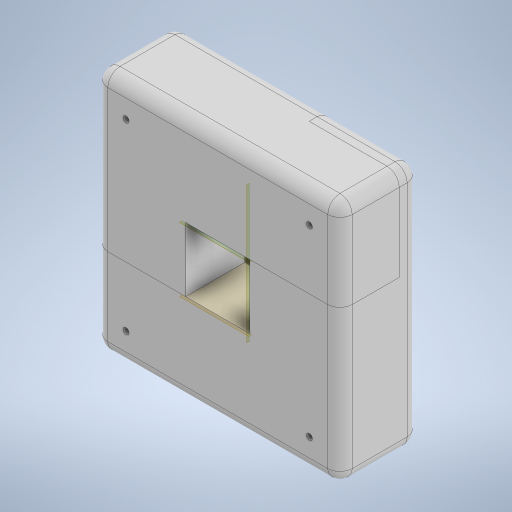
# Autodesk Inventor part: BGO-holder-C-conector
Saved by Autodesk Inventor 2023 (Build 270158000, 158)
## iProperties
Created: 2023-12-01
Part Number: BGO-holder-C-conector
Material: Generic
Document SubType Name: Modeling
Designer: AxLab
Density: 1 g/cm^3
Appearance: Default
Author: AxLab
Autodesk Inventor part; units mm, degrees
ref_plane "YZ Plane" through (0, 0, 0) normal (1, 0, 0) x (0, 1, 0)
ref_plane "XZ Plane" through (0, 0, 0) normal (0, 1, 0) x (-1, 0, 0)
ref_plane "XY Plane" through (0, 0, 0) normal (0, 0, 1) x (1, 0, 0)
sketch "Sketch1" plane through (0, 0, 0) normal (0, 0, 1) x (1, 0, 0)
  line L0 (-20, -20) -> (20, -20)
  line L1 (20, -20) -> (20, 20)
  line L2 (20, 20) -> (-20, 20)
  line L3 (-20, 20) -> (-20, -20)
  line L4 (-20, -20) -> (20, 20) construction
  line L5 (20, -20) -> (-20, 20) construction
  point P0 (0, 0)
  dimension "d0" = 40
  dimension "d1" = 40
  constraints: 12 end point, 2 midpoint, 2 parallel, 1 horizontal, 1 perpendicular
  measures "d0" distance of L2.end L1.end
  measures "d1" distance of L1.end L0.end
extrude "Extrusion1" add sketch "Sketch1" along normal blind 13
sketch "Sketch2" plane through (0, 0, 13) normal (0, 0, 1) x (1, 0, 0)
  line L0 (5.25, -5.25) -> (-5.25, -5.25)
  line L1 (-5.25, -5.25) -> (-5.25, 5.25)
  line L2 (-5.25, 5.25) -> (5.25, 5.25)
  line L3 (5.25, 5.25) -> (5.25, -5.25)
  line L4 (5.25, -5.25) -> (-5.25, 5.25) construction
  line L5 (-5.25, -5.25) -> (5.25, 5.25) construction
  point P0 (0, 0)
  dimension "d4" = 10.5
  dimension "d5" = 10.5
  constraints: 12 end point, 2 midpoint, 2 parallel, 1 horizontal, 1 perpendicular
  measures "d4" distance of L1.end L2.end
  measures "d5" distance of L0.end L1.end
extrude "Extrusion2" cut sketch "Sketch2" against normal blind 9.7
sketch "Sketch3" plane through (0, 0, 13) normal (0, 0, 1) x (1, 0, 0)
  line L0 (-20, 20) -> (-20, -20) projected
  line L1 (-20, 20) -> (-15, 20)
  line L2 (-15, 20) -> (-15, 15)
  line L3 (-15, 15) -> (-20, 15)
  line L4 (-20, 15) -> (-20, 20)
  circle A0 centre (-15, 15) radius 0.5
  point P0 (0, 0)
  dimension "d8" = 5
  dimension "d9" = 5
  dimension "d10" = 1
  constraints: 8 end point, 2 parallel, 1 centre point, 1 coincident, 1 horizontal, 1 perpendicular
  measures "d8" distance of L2.end L3.end
  measures "d9" distance of L1.end L2.end
  measures "d10" diameter of A0
extrude "Extrusion3" cut sketch "Sketch3" against normal blind 13 contours A0 L2 L3 | L3 L2 A0
mirror "Mirror1" about plane through (0, 0, 0) normal (0, 1, 0) of "Extrusion3"
mirror "Mirror2" about plane through (0, 0, 0) normal (1, 0, 0) of "Extrusion3", "Mirror1"
ref_plane "Work Plane1" through (-5.25, -5.25, 13) normal (0, 1, 0) x (1, 0, 0)
ref_plane "Work Plane2" through (-5.25, 5.25, 13) normal (0, -1, 0) x (1, 0, 0)
ref_plane "Work Plane3" through (5.25, -5.25, 13) normal (-1, 0, 0) x (0, 0, 1)
ref_plane "Work Plane4" through (0, 0, 3.3) normal (0, 0, 1) x (1, 0, 0)
split body "Split4" result two bodies by plane through (5.25, -5.25, 13) normal (-1, 0, 0) first body at (-1.3752, -4.8895, 0.5)
split body "Split5" result two bodies by plane through (-5.25, 5.25, 13) normal (0, -1, 0) bodies 3 first body at (13.3966, -1.3345, 0.5)
split body "Split6" result two bodies by plane through (-5.25, -5.25, 13) normal (0, 1, 0) bodies 2 first body at (-9.822, 1.3628, 0.5)
split body "Split7" result two bodies by plane through (0, 0, 3.3) normal (0, 0, 1) bodies 7 first body at (-4.8333, -13.4167, 3.8)
split body "Split8" result two bodies by plane through (0, 0, 3.3) normal (0, 0, 1) bodies 5 first body at (13.3576, 8.3442, 3.8)
combine bodies "Combine1" operation type add bodies to combine 11 4 8
combine bodies "Combine2" operation type add bodies to combine 10 6 9
fillet "Fillet2" radius 2 18 edges at (-20, 20, 6.5) (-20, 0, 0) (-20, -20, 1.65) (-20, 7.375, 13) (0, 20, 13) (-7.375, 20, 0) (20, 12.625, 13) (20, 20, 8.15) (-7.375, -20, 0) (-20, -20, 8.15) (0, -20, 13) (-20, -12.625, 13) (20, -7.375, 13) (20, -20, 6.5) (12.625, 20, 0) (20, 20, 1.65) (20, 0, 0) (12.625, -20, 0)
body "Solid10"
body "Solid11"
